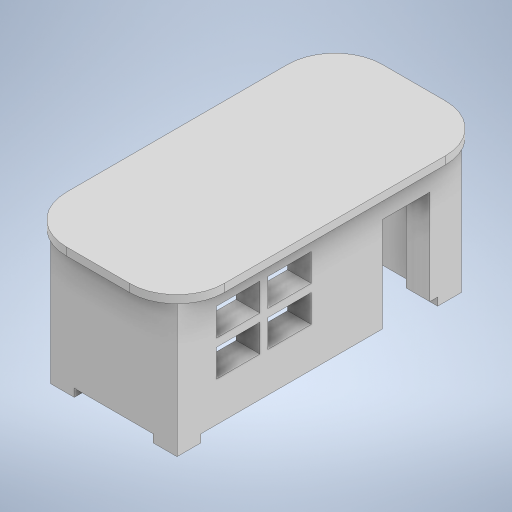
# Autodesk Inventor part: huis
Saved by Autodesk Inventor 2023 (Build 270158000, 158)
## iProperties
Created: 2023-06-06
Part Number: huis
Material: Generic
Document SubType Name: Modeling
Designer: Prestige
Density: 1 g/cm^3
Appearance: Default
Author: Prestige
Autodesk Inventor part; units mm, degrees
ref_plane "YZ Plane" through (0, 0, 0) normal (1, 0, 0) x (0, 1, 0)
ref_plane "XZ Plane" through (0, 0, 0) normal (0, 1, 0) x (-1, 0, 0)
ref_plane "XY Plane" through (0, 0, 0) normal (0, 0, 1) x (1, 0, 0)
sketch "Sketch1" plane through (0, 0, 0) normal (0, 1, 0) x (-1, 0, 0)
  line L0 (0, 0) -> (15, 0)
  line L1 (15, 0) -> (15, -15)
  line L2 (15, -15) -> (0, -15)
  line L3 (0, -15) -> (0, 0)
  line L4 (15, -165) -> (0, -165)
  line L5 (0, -165) -> (0, -180)
  line L6 (0, -180) -> (15, -180)
  line L7 (15, -180) -> (15, -165)
  line L8 (65, -180) -> (80, -180)
  line L9 (80, -180) -> (80, -165)
  line L10 (80, -165) -> (65, -165)
  line L11 (65, -165) -> (65, -180)
  line L12 (80, -15) -> (65, -15)
  line L13 (65, -15) -> (65, 0)
  line L14 (65, 0) -> (80, 0)
  line L15 (80, 0) -> (80, -15)
  point P0 (15, -7.5)
  dimension "d0" = 15
  dimension "d1" = 15
  dimension "d2" = 15
  dimension "d3" = 15
  dimension "d4" = 15
  dimension "d5" = 15
  dimension "d6" = 150
  dimension "d7" = 50
  constraints: 32 end point, 8 parallel, 7 point on line, 4 horizontal, 4 perpendicular, 1 midpoint
  measures "d0" distance of L12.start L12.end
  measures "d1" distance of L14.end L12.start
  measures "d2" distance of L9.end L10.end
  measures "d3" distance of L8.end L9.end
  measures "d4" distance of L5.end L6.end
  measures "d5" distance of L0.end L1.end
  measures "d6" distance between parallel lines of L12 L10
  measures "d7" distance from line of L13 point (15, -7.5)
extrude "Extrusion1" add sketch "Sketch1" along normal blind 5
sketch "Sketch2" plane through (0, 5, 0) normal (0, 1, 0) x (1, 0, 0)
  line L0 (-80, 0) -> (-65, 0) projected
  line L1 (-80, 0) -> (-65, 0)
  line L2 (-65, 0) -> (-65, 180)
  line L3 (-65, 180) -> (-80, 180)
  line L4 (-80, 180) -> (-80, 0)
  line L5 (-15, 165) -> (0, 165) projected
  line L6 (-65, 180) -> (0, 180)
  line L7 (0, 180) -> (0, 165)
  line L8 (0, 165) -> (-65, 165)
  line L9 (-65, 165) -> (-65, 180)
  line L10 (-15, 0) -> (0, 0) projected
  line L11 (-15, 165) -> (0, 165)
  line L12 (0, 165) -> (0, 0)
  line L13 (0, 0) -> (-15, 0)
  line L14 (-15, 0) -> (-15, 165)
  line L15 (-15, 0) -> (-65, 0)
  line L16 (-65, 0) -> (-65, 15)
  line L17 (-65, 15) -> (-15, 15)
  line L18 (-15, 15) -> (-15, 0)
  point P0 (-65, 165)
  constraints: 32 end point, 8 parallel, 4 horizontal, 4 perpendicular
extrude "Extrusion2" add sketch "Sketch2" along normal blind 80 contours L4 L3 L2 L0 | L2 L17 L14 L15 | L14 L5 L12 L10 | L6 L7 L5 L8 L2
sketch "Sketch3" plane through (0, 85, 0) normal (0, 1, 0) x (1, 0, 0)
  line L0 (-90, -10) -> (10, -10)
  line L1 (10, -10) -> (10, 190)
  line L2 (10, 190) -> (-90, 190)
  line L3 (-90, 190) -> (-90, -10)
  line L4 (-80, 180) -> (-80, 0) projected
  line L5 (0, 180) -> (-80, 180) projected
  line L6 (0, 0) -> (0, 180) projected
  line L7 (-80, 0) -> (0, 0) projected
  point P0 (-40, -10)
  dimension "d12" = 10
  dimension "d13" = 10
  dimension "d14" = 10
  dimension "d15" = 10
  constraints: 8 end point, 2 parallel, 1 horizontal, 1 midpoint, 1 perpendicular
  measures "d12" distance between parallel lines of L3 L4
  measures "d13" distance between parallel lines of L2 L5
  measures "d14" distance between parallel lines of L6 L1
  measures "d15" distance from line of L7 point (-40, -10)
extrude "Extrusion3" add sketch "Sketch3" along normal blind 5 contours L3 L2 L1 L0 | L5 L6 L7 L4
fillet "Fillet1" radius 30 4 edges at (10, 87.5, 10) (-90, 87.5, 10) (-90, 87.5, -190) (10, 87.5, -190)
sketch "Sketch4" plane through (0, 0, 0) normal (1, 0, 0) x (0, 0, -1)
  line L0 (160, 5) -> (130, 5)
  line L1 (130, 5) -> (130, 65)
  line L2 (130, 65) -> (160, 65)
  line L3 (160, 65) -> (160, 5)
  line L4 (25, 70) -> (85, 70)
  line L5 (85, 70) -> (85, 30)
  line L6 (85, 30) -> (25, 30)
  line L7 (25, 30) -> (25, 70)
  line L8 (0, 0) -> (0, 85) projected
  line L9 (180, 0) -> (180, 85) projected
  line L10 (15, 5) -> (165, 5) projected
  line L11 (20, 85) -> (160, 85) projected
  line L12 (52.5, 70) -> (57.5, 70)
  line L13 (57.5, 70) -> (57.5, 30)
  line L14 (57.5, 30) -> (52.5, 30)
  line L15 (52.5, 30) -> (52.5, 70)
  line L16 (85, 52.5) -> (25, 52.5)
  line L17 (25, 52.5) -> (25, 47.5)
  line L18 (25, 47.5) -> (85, 47.5)
  line L19 (85, 47.5) -> (85, 52.5)
  point P0 (52.5, 52.5)
  point P1 (52.5, 47.5)
  point P2 (57.5, 47.5)
  point P3 (57.5, 52.5)
  dimension "d19" = 60
  dimension "d20" = 30
  dimension "d21" = 40
  dimension "d22" = 60
  dimension "d23" = 25
  dimension "d24" = 20
  dimension "d25" = 0
  dimension "d26" = 15
  dimension "d27" = 5
  dimension "d28" = 5
  dimension "d29" = 17.5
  dimension "d30" = 27.5
  constraints: 32 end point, 8 parallel, 4 horizontal, 4 perpendicular, 4 point on line
  measures "d19" distance of L2.end L0.start
  measures "d20" distance of L1.end L2.end
  measures "d21" distance of L4.end L5.end
  measures "d22" distance of L4.start L4.end
  measures "d23" distance between parallel lines of L8 L7
  measures "d24" distance between parallel lines of L9 L3
  measures "d25" distance between parallel lines of L10 L0
  measures "d26" distance between parallel lines of L11 L4
  measures "d27" distance between parallel lines of L15 L13
  measures "d28" distance between parallel lines of L18 L16
  measures "d29" distance between parallel lines of L4 L16
  measures "d30" distance between parallel lines of L5 L13
extrude "Extrusion4" cut sketch "Sketch4" against normal blind 15 contours L0 L1 L2 L3 | L4 L15 L16 L7 | L4 L5 L16 L13 | L18 L15 L6 L7 | L18 L5 L6 L13
body "Solid1"
